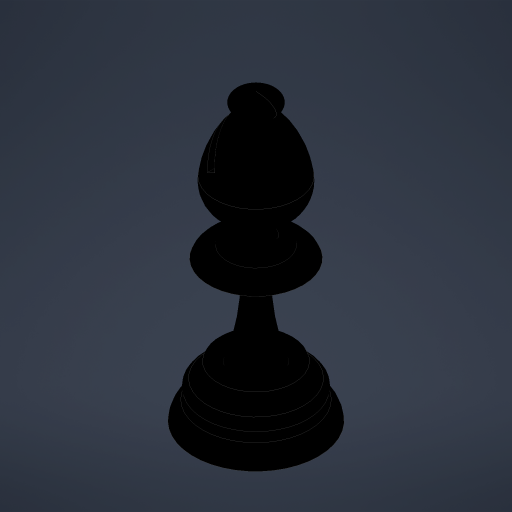
# Autodesk Inventor part: střelec černý
Saved by Autodesk Inventor 2023 (Build 270158000, 158)
## iProperties
Created: 2023-04-21
Part Number: střelec černý
Material: Generic
Document SubType Name: Modeling
Designer: X-DIABLO
Density: 1 g/cm^3
Appearance: Default
Author: X-DIABLO
Autodesk Inventor part; units mm, degrees
ref_plane "YZ Plane" through (0, 0, 0) normal (1, 0, 0) x (0, 1, 0)
ref_plane "XZ Plane" through (0, 0, 0) normal (0, 1, 0) x (-1, 0, 0)
ref_plane "XY Plane" through (0, 0, 0) normal (0, 0, 1) x (1, 0, 0)
sketch "Sketch1" plane through (0, 0, 0) normal (0, 0, 1) x (1, 0, 0)
  arc A0 (10.6154, 14.4572) -> (6.4844, 14.3615) centre (8.5595, 13.9943) ccw
  arc A1 (10.6154, 14.4572) -> (13.3879, 10.3297) centre (17.3221, 15.9672) ccw
  arc A2 (14.5003, 7.5665) -> (13.3879, 10.3297) centre (12.7286, 8.4588) ccw
  arc A3 (17.5, 0) -> (14.9429, 5.1854) centre (9.655, -0.6454) ccw
  arc A4 (14.5003, 7.5665) -> (14.9429, 5.1854) centre (16.2865, 6.6669) ccw
  line L0 (0, 0) -> (0, 80)
  arc A5 (4.2116, 50.1216) -> (11.5396, 59.4813) centre (3.2387, 58.4318) ccw
  ellipse E0 centre (0, 48.2376) end of major axis (6.4661, 48.2376) minor radius 2.483 (4.6364, 46.5068) -> (4.2116, 50.1216) ccw
  arc A6 (8.0438, 42.7386) -> (4.6364, 46.5068) centre (4.6136, 43.0616) ccw
  line L1 (3.2611, 39.4908) -> (13.1972, 39.4908)
  arc A7 (3.2611, 39.4908) -> (6.4844, 14.3615) centre (64.376, 34.5586) ccw
  arc A8 (13.1972, 39.4908) -> (8.0438, 42.7386) centre (8.7166, 38.0938) ccw
  line L2 (17.5, 0) -> (0, 0)
  ellipse E1 centre (0, 77.3248) end of major axis (5.7122, 77.3248) minor radius 2.6752 (3.5629, 75.2337) -> (0, 80) ccw
  arc A9 (11.5396, 59.4813) -> (3.5629, 75.2337) centre (-14.5057, 56.1884) ccw
  point P0 (0, 0)
  dimension "d0" = 2
  dimension "d1" = 80
  constraints: 20 point on circle, 10 centre point, 6 end point, 4 tangent, 2 point on line, 2 vertical, 1 horizontal, 1 perpendicular, 8 other
  measures "d0" radius of A4
  measures "d1" distance of L0.end L0.start
revolve "Revolution1" add sketch "Sketch1" angle 360 about axis through (0, 0, 0) along (0, 1, 0)
sketch "Sketch2" plane through (0, 0, 0) normal (0, 0, 1) x (1, 0, 0)
  line L0 (3.5629, 75.2337) -> (-3.5629, 75.2337) projected
  line L1 (11.5396, 59.4813) -> (-11.5396, 59.4813) projected
  line L2 (-9.366, 75.2337) -> (-3.5629, 63.5627)
  line L3 (-3.5629, 63.5627) -> (-1.3243, 64.6757)
  line L4 (-1.3243, 64.6757) -> (-7.1274, 76.3468)
  line L5 (-7.1274, 76.3468) -> (-9.366, 75.2337)
  point P0 (0, 0)
  dimension "d3" = 2.5
  constraints: 8 end point, 3 perpendicular
  measures "d3" distance of L2.end L3.end
extrude "Extrusion1" cut sketch "Sketch2" along normal mid plane 100
body "Solid1"
